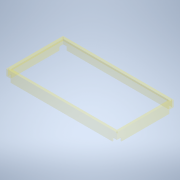
# Autodesk Inventor part: FINAL 2X2 FABRIC
Saved by Autodesk Inventor 2022 (Build 260153000, 153)
## iProperties
Created: 2021-08-25
Part Number: FINAL 2X2 FABRIC
Material: Generic
Document SubType Name: Modeling
Designer: benka
Density: 1 g/cm^3
Appearance: Clear - Yellow
Author: benka
Autodesk Inventor part; units mm, degrees
ref_plane "YZ Plane" through (0, 0, 0) normal (1, 0, 0) x (0, 1, 0)
ref_plane "XZ Plane" through (0, 0, 0) normal (0, 1, 0) x (-1, 0, 0)
ref_plane "XY Plane" through (0, 0, 0) normal (0, 0, 1) x (1, 0, 0)
sketch "Sketch1" plane through (0, 0, 0) normal (0, 1, 0) x (-1, 0, 0)
  line L0 (-173, 86) -> (150.0804, 86)
  line L1 (173, -86) -> (-173, -86)
  line L2 (150.0804, 86) -> (173, 86)
  line L3 (-175, -84) -> (-175, 84)
  line L4 (175, 84) -> (175, -84)
  arc A0 (-173, 86) -> (-175, 84) centre (-173, 84) ccw
  arc A1 (-175, -84) -> (-173, -86) centre (-173, -84) ccw
  arc A2 (173, -86) -> (175, -84) centre (173, -84) ccw
  arc A3 (175, 84) -> (173, 86) centre (173, 84) ccw
  circle A4 centre (-179, 90) radius 1.5
  circle A5 centre (179, 90) radius 1.5
  line L5 (0, 0) -> (-13.5722, 0)
  circle A6 centre (-179, -90) radius 1.5
  circle A7 centre (179, -90) radius 1.5
  line L6 (0, 0) -> (0, -14.8984)
  line L7 (183, -64.0758) -> (180, -64.0758)
  line L8 (180, -64.0758) -> (180, -32.8017)
  line L9 (180, -32.8017) -> (183, -32.8017)
  line L10 (180, 64.0758) -> (180, 32.8017)
  line L11 (180, 32.8017) -> (183, 32.8017)
  line L12 (180, 0) -> (180, -10)
  line L13 (180, -10) -> (183, -10)
  line L14 (183, 10) -> (180, 10)
  line L15 (180, 10) -> (180, 0)
  line L16 (180, 64.0758) -> (183, 64.0758)
  line L17 (-183, -64.0758) -> (-180, -64.0758)
  line L18 (-180, -64.0758) -> (-180, -32.8017)
  line L19 (-180, -32.8017) -> (-183, -32.8017)
  line L20 (-180, 64.0758) -> (-180, 32.8017)
  line L21 (-180, 32.8017) -> (-183, 32.8017)
  line L22 (-180, 0) -> (-180, -10)
  line L23 (-180, -10) -> (-183, -10)
  line L24 (-183, 10) -> (-180, 10)
  line L25 (-180, 10) -> (-180, 0)
  line L26 (-180, 64.0758) -> (-183, 64.0758)
  line L27 (115.3851, 94) -> (115.3851, 91)
  line L28 (115.3851, 91) -> (165.3851, 91)
  line L29 (165.3851, 91) -> (165.3851, 94)
  line L30 (50, 94) -> (50, 91)
  line L31 (50, 91) -> (0, 91)
  line L32 (-115.3851, 94) -> (-115.3851, 91)
  line L33 (-115.3851, 91) -> (-165.3851, 91)
  line L34 (-165.3851, 91) -> (-165.3851, 94)
  line L35 (-50, 94) -> (-50, 91)
  line L36 (-50, 91) -> (0, 91)
  line L37 (115.3851, -94) -> (115.3851, -91)
  line L38 (115.3851, -91) -> (165.3851, -91)
  line L39 (165.3851, -91) -> (165.3851, -94)
  line L40 (50, -94) -> (50, -91)
  line L41 (50, -91) -> (0, -91)
  line L42 (-50, -94) -> (-50, -91)
  line L43 (-50, -91) -> (0, -91)
  line L44 (-115.3851, -94) -> (-115.3851, -91)
  line L45 (-115.3851, -91) -> (-165.3851, -91)
  line L46 (-165.3851, -91) -> (-165.3851, -94)
  line L47 (183, -94) -> (183, -64.0758)
  line L48 (183, -32.8017) -> (183, -10)
  line L49 (183, 10) -> (183, 32.8017)
  line L50 (183, 64.0758) -> (183, 94)
  line L51 (-50, 94) -> (-115.3851, 94)
  line L52 (-165.3851, 94) -> (-183, 94)
  line L53 (183, 94) -> (165.3851, 94)
  line L54 (115.3851, 94) -> (50, 94)
  line L55 (-183, 94) -> (-183, 64.0758)
  line L56 (-183, 32.8017) -> (-183, 10)
  line L57 (-183, -10) -> (-183, -32.8017)
  line L58 (-183, -64.0758) -> (-183, -94)
  line L59 (-183, -94) -> (-165.3851, -94)
  line L60 (-115.3851, -94) -> (-50, -94)
  line L61 (50, -94) -> (115.3851, -94)
  line L62 (165.3851, -94) -> (183, -94)
  point P0 (0, 0)
  point P1 (175, -86)
  point P2 (-175, -86)
  dimension "d0" = 172
  dimension "d1" = 350
  dimension "d2" = 2
  dimension "d3" = 175
  dimension "d4" = 175
  dimension "d5" = 350
  dimension "d6" = 86
  dimension "d9" = 3
  constraints: 126 end point, 37 symmetric about line, 8 centre point, 8 point on circle, 8 tangent, 5 perpendicular, 4 point on line, 3 equal radius, 3 horizontal, 3 parallel, 2 vertical, 2 other
  measures "d0" distance between parallel lines of L1 L0
  measures "d1" distance of point (175, -86) point (-175, -86)
  measures "d2" radius of A0
  measures "d3" distance from line of L5.start L3
  measures "d4" distance from line of L4 L5.start
  measures "d5" distance between parallel lines of L4 L3
  measures "d6" distance from line of L5.start L1
  measures "d9" diameter of A4
extrude "Extrusion1" add sketch "Sketch1" along normal blind 3
sketch "Sketch3" plane through (-165.3851, 0, 91) normal (0, 0, 1) x (1, 0, 0)
  line L0 (-14.6149, -15.0793) -> (-4.6149, -15.0793)
  line L1 (-2.6149, -17.0793) -> (-2.6149, -27)
  line L2 (333.3851, -27) -> (333.3851, -17.0793)
  line L3 (335.3851, -15.0793) -> (345.3851, -15.0793)
  line L4 (-17.6149, 0) -> (0, 0) projected
  line L5 (0, 0) -> (0, 3) projected
  line L6 (0, 3) -> (50, 3) projected
  line L7 (50, 0) -> (50, 3) projected
  line L8 (50, 0) -> (115.3851, 0) projected
  line L9 (115.3851, 0) -> (115.3851, 3) projected
  line L10 (115.3851, 3) -> (215.3851, 3) projected
  line L11 (215.3851, 0) -> (215.3851, 3) projected
  line L12 (215.3851, 0) -> (280.7703, 0) projected
  line L13 (280.7703, 0) -> (280.7703, 3) projected
  line L14 (280.7703, 3) -> (330.7703, 3) projected
  line L15 (330.7703, 0) -> (330.7703, 3) projected
  line L16 (330.7703, 0) -> (348.3851, 0) projected
  line L17 (-2.6149, -27) -> (333.3851, -27)
  arc A0 (-2.6149, -17.0793) -> (-4.6149, -15.0793) centre (-4.6149, -17.0793) ccw
  arc A1 (335.3851, -15.0793) -> (333.3851, -17.0793) centre (335.3851, -17.0793) ccw
  line L18 (348.3851, -8.5793) -> (348.3851, 0)
  line L19 (-17.6149, 0) -> (-17.6149, 3) projected
  line L20 (-17.6149, -8.5793) -> (-17.6149, 0)
  line L21 (-17.6149, -8.5793) -> (-14.6149, -8.5793)
  line L22 (-14.6149, -8.5793) -> (-14.6149, -15.0793)
  line L23 (345.3851, -8.5793) -> (348.3851, -8.5793)
  line L24 (345.3851, -15.0793) -> (345.3851, -8.5793)
  point P0 (165.3851, 0)
  dimension "d37" = 30
  dimension "d39" = 2
  constraints: 22 end point, 4 point on circle, 4 tangent, 3 horizontal, 2 centre point, 2 vertical, 1 equal radius, 1 perpendicular
  measures "d37" distance between parallel lines of L6 L17
  measures "d39" radius of A0
extrude "Extrusion2" add sketch "Sketch3" along normal blind 3
sketch "Sketch4" plane through (305.7703, 13.5, -91) normal (0, 0, -1) x (-1, 0, 0)
  line L0 (125.7703, -28.5793) -> (135.7703, -28.5793)
  line L1 (137.7703, -30.5793) -> (137.7703, -40.5)
  line L2 (473.7703, -40.5) -> (473.7703, -30.5793)
  line L3 (475.7703, -28.5793) -> (485.7703, -28.5793)
  line L4 (122.7703, -13.5) -> (140.3851, -13.5)
  line L5 (140.3851, -13.5) -> (140.3851, -10.5)
  line L6 (140.3851, -10.5) -> (190.3851, -10.5)
  line L7 (190.3851, -13.5) -> (190.3851, -10.5)
  line L8 (190.3851, -13.5) -> (255.7703, -13.5)
  line L9 (255.7703, -13.5) -> (255.7703, -10.5)
  line L10 (255.7703, -10.5) -> (355.7703, -10.5)
  line L11 (355.7703, -13.5) -> (355.7703, -10.5)
  line L12 (355.7703, -13.5) -> (421.1554, -13.5)
  line L13 (421.1554, -13.5) -> (421.1554, -10.5)
  line L14 (421.1554, -10.5) -> (471.1554, -10.5)
  line L15 (471.1554, -13.5) -> (471.1554, -10.5)
  line L16 (471.1554, -13.5) -> (488.7703, -13.5)
  line L17 (137.7703, -40.5) -> (473.7703, -40.5)
  arc A0 (137.7703, -30.5793) -> (135.7703, -28.5793) centre (135.7703, -30.5793) ccw
  arc A1 (475.7703, -28.5793) -> (473.7703, -30.5793) centre (475.7703, -30.5793) ccw
  line L18 (488.7703, -22.0793) -> (488.7703, -13.5)
  line L19 (122.7703, -22.0793) -> (122.7703, -13.5)
  line L20 (122.7703, -22.0793) -> (125.7703, -22.0793)
  line L21 (125.7703, -22.0793) -> (125.7703, -28.5793)
  line L22 (485.7703, -22.0793) -> (488.7703, -22.0793)
  line L23 (485.7703, -28.5793) -> (485.7703, -22.0793)
  dimension "d49" = 30
  dimension "d50" = 2
  constraints: 48 end point, 4 point on circle, 4 tangent, 3 horizontal, 2 centre point, 2 vertical, 1 equal radius, 1 perpendicular
  measures "d49" distance between parallel lines of L6 L17
  measures "d50" radius of A0
extrude "Extrusion4" add sketch "Sketch4" along normal blind 3
sketch "Sketch5" plane through (-180, 0, -64.0758) normal (-1, 0, 0) x (0, 0, 1)
  line L0 (-29.9242, -15.0793) -> (-29.9242, -8.5793) projected
  line L1 (-26.9242, -8.5793) -> (-29.9242, -8.5793) projected
  line L2 (-26.9242, -8.5793) -> (-26.9242, 0) projected
  line L3 (-26.9242, 0) -> (0, 0) projected
  line L4 (0, 0) -> (0, 3) projected
  line L5 (0, 3) -> (31.2741, 3) projected
  line L6 (31.2741, 0) -> (31.2741, 3) projected
  line L7 (54.0758, 0) -> (54.0758, 3) projected
  line L8 (54.0758, 3) -> (74.0758, 3) projected
  line L9 (31.2741, 0) -> (54.0758, 0) projected
  line L10 (74.0758, 0) -> (96.8775, 0) projected
  line L11 (96.8775, 0) -> (96.8775, 3) projected
  line L12 (74.0758, 0) -> (74.0758, 3) projected
  line L13 (96.8775, 3) -> (128.1515, 3) projected
  line L14 (128.1515, 0) -> (128.1515, 3) projected
  line L15 (128.1515, 0) -> (155.0758, 0) projected
  line L16 (155.0758, 0) -> (155.0758, -8.5793) projected
  line L17 (155.0758, -8.5793) -> (158.0758, -8.5793) projected
  line L18 (158.0758, -8.5793) -> (158.0758, -15.0793) projected
  line L19 (155.0758, -15.0793) -> (158.0758, -15.0793) projected
  line L20 (-26.9242, -15.0793) -> (-29.9242, -15.0793) projected
  line L21 (-26.9242, -15.0793) -> (-16.9242, -15.0793)
  line L22 (-14.9242, -17.0793) -> (-14.9242, -27)
  line L23 (155.0758, -15.0793) -> (158.0758, -15.0793) projected
  line L24 (155.0758, -15.0793) -> (145.0758, -15.0793)
  line L25 (143.0758, -17.0793) -> (143.0758, -27)
  line L26 (-14.9242, -27) -> (143.0758, -27)
  arc A0 (-14.9242, -17.0793) -> (-16.9242, -15.0793) centre (-16.9242, -17.0793) ccw
  arc A1 (145.0758, -15.0793) -> (143.0758, -17.0793) centre (145.0758, -17.0793) ccw
  point P0 (64.0758, 0)
  point P1 (-14.9242, -15.0793)
  point P2 (143.0758, -15.0793)
  dimension "d66" = 12
  dimension "d67" = 12
  dimension "d68" = 2
  constraints: 10 end point, 4 point on circle, 4 point on line, 4 tangent, 3 horizontal, 2 centre point, 1 equal radius, 1 perpendicular, 1 vertical
  measures "d66" distance of L20.start point (-14.924, -15.079)
  measures "d67" distance of L19.start point (143.076, -15.079)
  measures "d68" radius of A0
extrude "Extrusion5" add sketch "Sketch5" along normal blind 3
sketch "Sketch6" plane through (180, 0, 64.0758) normal (1, 0, 0) x (0, 0, -1)
  line L0 (-29.9242, -15.0793) -> (-29.9242, -8.5793)
  line L1 (-26.9242, -8.5793) -> (-29.9242, -8.5793)
  line L2 (-26.9242, -8.5793) -> (-26.9242, 0)
  line L3 (-26.9242, 0) -> (0, 0)
  line L4 (0, 0) -> (0, 3)
  line L5 (0, 3) -> (31.2741, 3)
  line L6 (31.2741, 0) -> (31.2741, 3)
  line L7 (54.0758, 0) -> (54.0758, 3)
  line L8 (54.0758, 3) -> (74.0758, 3)
  line L9 (31.2741, 0) -> (54.0758, 0)
  line L10 (74.0758, 0) -> (96.8775, 0)
  line L11 (96.8775, 0) -> (96.8775, 3)
  line L12 (74.0758, 0) -> (74.0758, 3)
  line L13 (96.8775, 3) -> (128.1515, 3)
  line L14 (128.1515, 0) -> (128.1515, 3)
  line L15 (128.1515, 0) -> (155.0758, 0)
  line L16 (155.0758, 0) -> (155.0758, -8.5793)
  line L17 (155.0758, -8.5793) -> (158.0758, -8.5793)
  line L18 (158.0758, -8.5793) -> (158.0758, -15.0793)
  line L19 (155.0758, -15.0793) -> (158.0758, -15.0793)
  line L20 (-26.9242, -15.0793) -> (-29.9242, -15.0793)
  line L21 (-26.9242, -15.0793) -> (-16.9242, -15.0793)
  line L22 (-14.9242, -17.0793) -> (-14.9242, -27)
  line L23 (155.0758, -15.0793) -> (158.0758, -15.0793)
  line L24 (155.0758, -15.0793) -> (145.0758, -15.0793)
  line L25 (143.0758, -17.0793) -> (143.0758, -27)
  line L26 (-14.9242, -27) -> (143.0758, -27)
  arc A0 (-14.9242, -17.0793) -> (-16.9242, -15.0793) centre (-16.9242, -17.0793) ccw
  arc A1 (145.0758, -15.0793) -> (143.0758, -17.0793) centre (145.0758, -17.0793) ccw
  point P0 (64.0758, 0)
  point P1 (64.0758, 0)
  point P2 (-14.9242, -15.0793)
  point P3 (143.0758, -15.0793)
  dimension "d71" = 12
  dimension "d72" = 12
  dimension "d73" = 2
  constraints: 54 end point, 4 point on circle, 4 point on line, 4 tangent, 3 horizontal, 2 centre point, 1 equal radius, 1 perpendicular, 1 vertical
  measures "d71" distance of L21.start point (-14.924, -15.079)
  measures "d72" distance of L24.start point (143.076, -15.079)
  measures "d73" radius of A0
extrude "Extrusion6" add sketch "Sketch6" along normal blind 3
sketch "Sketch2" plane through (0, 0, 0) normal (0, 1, 0) x (-1, 0, 0)
  line L0 (-175, -84) -> (-175, 84)
  line L1 (-183, 94) -> (-183, -94)
  line L2 (0, -94) -> (-8.1698, -94)
  line L3 (183, 94) -> (-183, 94)
  line L4 (173, -86) -> (-173, -86)
  line L5 (-183, -94) -> (183, -94)
  line L6 (183, -94) -> (183, 94)
  line L7 (-173, 86) -> (150.0804, 86)
  arc A0 (-173, 86) -> (-175, 84) centre (-173, 84) ccw
  circle A1 centre (-179, 90) radius 1.5
  arc A2 (-175, -84) -> (-173, -86) centre (-173, -84) ccw
  arc A3 (175, 84) -> (173, 86) centre (173, 84) ccw
  arc A4 (173, -86) -> (175, -84) centre (173, -84) ccw
  line L8 (175, 84) -> (175, -84)
  line L9 (150.0804, 86) -> (173, 86)
  circle A5 centre (179, 90) radius 1.5
  line L10 (0, 0) -> (-13.5722, 0)
  circle A6 centre (179, -90) radius 1.5
  circle A7 centre (-179, -90) radius 1.5
  point P0 (0, 0)
  point P1 (0, 0)
  point P2 (-175, -86)
  point P3 (175, -86)
  dimension "d12" = 172
  dimension "d13" = 350
  dimension "d14" = 2
  dimension "d15" = 175
  dimension "d16" = 175
  dimension "d17" = 350
  dimension "d18" = 86
  dimension "d19" = 8
  dimension "d20" = 8
  dimension "d21" = 3
  dimension "d22" = 4
  dimension "d23" = 4
  constraints: 22 end point, 8 centre point, 8 point on circle, 8 tangent, 4 point on line, 3 equal radius, 3 horizontal, 2 symmetric about line, 1 parallel, 1 vertical, 2 other
  measures "d12" distance between parallel lines of L4 L7
  measures "d13" distance of point (175, -86) point (-175, -86)
  measures "d14" radius of A0
  measures "d15" distance from line of L10.start L0
  measures "d16" distance from line of L8 L10.start
  measures "d17" distance between parallel lines of L8 L0
  measures "d18" distance from line of L10.start L4
  measures "d19" distance between parallel lines of L0 L1
  measures "d20" distance between parallel lines of L3 L7
  measures "d21" diameter of A1
  measures "d22" distance from line of L1 A1.centre
  measures "d23" distance from line of A1.centre L3
sketch "Sketch7" plane through (0, 3, 0) normal (0, 1, 0) x (1, 0, 0)
  line L0 (183, 94) -> (-183, 94) projected
  line L1 (-183, 94) -> (-183, -94) projected
  line L2 (-183, -94) -> (183, -94) projected
  line L3 (183, -94) -> (183, 94) projected
  circle A0 centre (179, -90) radius 1.5 projected
  circle A1 centre (-179, -90) radius 1.5 projected
  circle A2 centre (-179, 90) radius 1.5 projected
  circle A3 centre (179, 90) radius 1.5 projected
  line L4 (-173, 86) -> (173, 86) projected
  arc A4 (175, 84) -> (173, 86) centre (173, 84) ccw projected
  line L5 (175, 84) -> (175, -84) projected
  arc A5 (173, -86) -> (175, -84) centre (173, -84) ccw projected
  line L6 (173, -86) -> (-173, -86) projected
  arc A6 (-175, -84) -> (-173, -86) centre (-173, -84) ccw projected
  line L7 (-175, -84) -> (-175, 84) projected
  arc A7 (-173, 86) -> (-175, 84) centre (-173, 84) ccw projected
  point P0 (0, 0)
extrude "Extrusion7" add sketch "Sketch7" along normal blind 3
body "Solid1"
